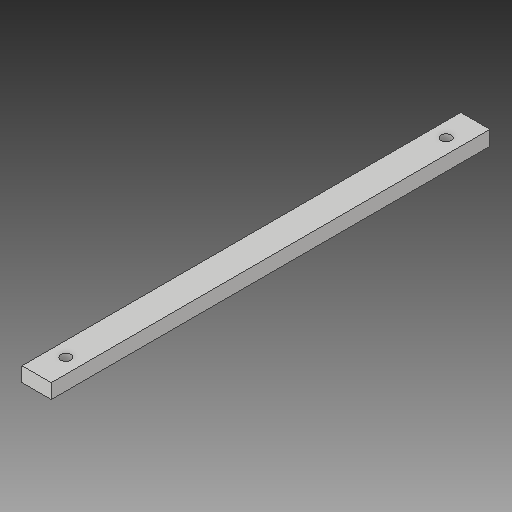
# Autodesk Inventor part: Arms
Saved by Autodesk Inventor 2019 (Build 230136000, 136)
## iProperties
Created: 2019-09-29
Part Number: Arms
Material: Generic
Document SubType Name: Modeling
Designer: james
Density: 1 g/cm^3
Appearance: Default
Mass: 0.970611 g
Surface Area: 12.0554 cm^2
Volume: 0.970611 cm^3
Author: james
Autodesk Inventor part; units mm, degrees
ref_plane "YZ Plane" through (0, 0, 0) normal (1, 0, 0) x (0, 1, 0)
ref_plane "XZ Plane" through (0, 0, 0) normal (0, 1, 0) x (-1, 0, 0)
ref_plane "XY Plane" through (0, 0, 0) normal (0, 0, 1) x (1, 0, 0)
sketch "Sketch1" plane through (0, 0, 0) normal (0, 1, 0) x (-1, 0, 0)
  line L0 (9.9449, 30.2649) -> (4.8649, 30.2649)
  line L1 (4.8649, 30.2649) -> (4.8649, -45.9351)
  line L2 (4.8649, -45.9351) -> (9.9449, -45.9351)
  line L3 (9.9449, -45.9351) -> (9.9449, 30.2649)
  point P0 (0, 0)
  dimension "d0" = 76.2
  dimension "d1" = 5.08
  constraints: 8 end point, 2 parallel, 1 horizontal, 1 perpendicular
  measures "d0" distance of L0.end L1.end
  measures "d1" distance of L0.start L0.end
extrude "Extrusion1" add sketch "Sketch1" along normal blind 2.54
sketch "Sketch2" plane through (0, 2.54, 0) normal (0, 1, 0) x (1, 0, 0)
  line L0 (-9.9449, -30.2649) -> (-4.8649, -30.2649) projected
  line L1 (-9.9449, 45.9351) -> (-9.9449, -30.2649) projected
  line L2 (-4.8649, 45.9351) -> (-9.9449, 45.9351) projected
  point P0 (0, 0)
  point P1 (-7.4049, -25.1849)
  point P2 (-7.4049, 40.8551)
  dimension "d4" = 5.08
  dimension "d5" = 2.54
  dimension "d6" = 2.54
  dimension "d7" = 5.08
  measures "d4" distance from line of L0 point (-7.405, -25.185)
  measures "d5" distance from line of L1 point (-7.405, -25.185)
  measures "d6" distance from line of L1 point (-7.405, 40.855)
  measures "d7" distance from line of L2 point (-7.405, 40.855)
hole "Hole1" at (-7.4049, 2.54, 25.1849) at (-7.4049, 2.54, -40.8551) direction (0, -1, 0) diameter 1.778 end through all
body "Solid1"
